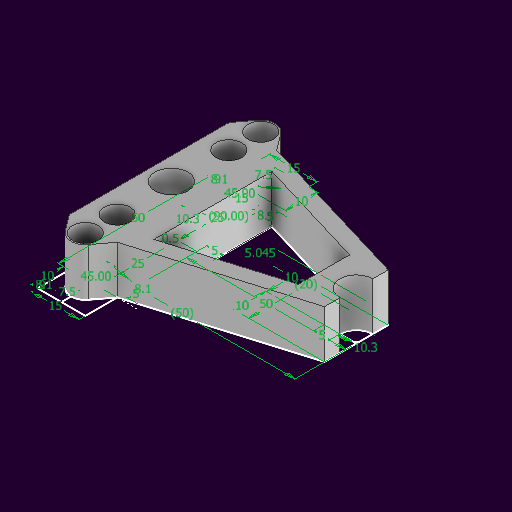
# Autodesk Inventor part: Rod_support_2.1
Saved by Autodesk Inventor 2026.2 (Build 302298000, 298)
## iProperties
Created: 2025-12-19
Part Number: Rod_support_2.1
Material: Generic
Document SubType Name: Modeling
Designer: Cobble
Density: 1 g/cm^3
Appearance: Default
Author: Cobble
Autodesk Inventor part; units mm, degrees
ref_plane "YZ Plane" through (0, 0, 0) normal (1, 0, 0) x (0, 1, 0)
ref_plane "XZ Plane" through (0, 0, 0) normal (0, 1, 0) x (-1, 0, 0)
ref_plane "XY Plane" through (0, 0, 0) normal (0, 0, 1) x (1, 0, 0)
sketch "Sketch1" plane through (0, 0, 0) normal (0, 0, 1) x (1, 0, 0)
  arc A0 (65, 30.15) -> (65, 19.85) centre (65, 25) ccw
  line L0 (65, 30.15) -> (65, 35)
  line L1 (65, 19.85) -> (65, 15)
  line L2 (65, 25) -> (15, 25)
  line L3 (15, 25) -> (15, 50)
  line L4 (15, 25) -> (15, 0)
  line L5 (15, 0) -> (65, 15)
  line L6 (15, 50) -> (65, 35)
  line L7 (15, 50) -> (0, 50)
  line L8 (0, 50) -> (0, 0)
  line L9 (0, 0) -> (15, 0)
  line L10 (15, 25) -> (20, 25)
  line L11 (20, 25) -> (20, 48.5)
  line L12 (20, 25) -> (20, 1.5)
  line L13 (59.85, 25) -> (54.85, 25)
  line L14 (54.85, 25) -> (54.85, 38.045)
  line L15 (54.85, 25) -> (54.85, 11.955)
  line L16 (20, 1.5) -> (20, 6.5)
  line L17 (20, 6.5) -> (54.85, 16.955)
  line L18 (20, 48.5) -> (20, 43.5)
  line L19 (20, 43.5) -> (54.85, 33)
  line L20 (7.5, 50) -> (7.5, 0)
  line L21 (0, 25) -> (15, 25)
  line L22 (0, 50) -> (15, 35)
  line L23 (0, 50) -> (21.2132, 50) construction
  line L24 (0, 0) -> (15, 15)
  line L25 (0, 0) -> (21.2132, 0) construction
  circle A1 centre (7.5, 7.5) radius 4.05
  circle A2 centre (7.5, 42.5) radius 4.05
  line L26 (65, 19.85) -> (65, 25)
  line L27 (65, 30.15) -> (65, 25)
  line L28 (7.5, 25) -> (7, 25)
  circle A3 centre (7, 25) radius 5.15
  line L29 (0, 50) -> (15, 50)
  line L30 (15, 50) -> (15, 60)
  line L31 (15, 60) -> (0, 60)
  line L32 (0, 60) -> (0, 50)
  line L33 (15, 0) -> (0, 0)
  line L34 (0, 0) -> (0, -10)
  line L35 (0, -10) -> (15, -10)
  line L36 (15, -10) -> (15, 0)
  line L37 (7.5, -10) -> (7.5, -2.5)
  line L38 (7.5, 60) -> (7.5, 52.5)
  circle A4 centre (7.5, 52.5) radius 4.05
  circle A5 centre (7.5, 52.5) radius 4.5
  circle A6 centre (7.5, -2.5) radius 4.05
  circle A7 centre (7.5, -2.5) radius 4.5
  line L39 (0, 50) -> (3.9, 55.2)
  line L40 (15, 50) -> (11.1, 55.2)
  line L41 (0, 0) -> (3.9, -5.2)
  line L42 (15, 0) -> (11.1, -5.2)
  point P0 (0, 0)
  point P1 (3.7583, 0)
  point P2 (11.2417, 0)
  point P3 (11.2417, 50)
  point P4 (3.7583, 50)
  point P5 (0, 0)
  dimension "d0" = 10.3
  dimension "d1" = 50
  dimension "d2" = 25
  dimension "d3" = 25
  dimension "d4" = 15
  dimension "d5" = 50
  dimension "d6" = 90
  dimension "d7" = 5
  dimension "d8" = 5
  dimension "d9" = 5
  dimension "d10" = 5
  dimension "d11" = 45
  dimension "d12" = 45
  dimension "d13" = 8.1
  dimension "d14" = 8.1
  dimension "d15" = 50
  dimension "d16" = 10
  dimension "d17" = 20
  dimension "d18" = 10
  dimension "d19" = 5.045
  dimension "d46" = 0.5
  dimension "d47" = 10.3
  dimension "d48" = 15
  dimension "d49" = 10
  dimension "d50" = 15
  dimension "d51" = 10
  dimension "d52" = 7.5
  dimension "d53" = 7.5
  dimension "d54" = 8.1
  dimension "d55" = 9
  dimension "d56" = 8.1
  dimension "d57" = 9
  constraints: 86 end point, 16 point on line, 8 centre point, 8 midpoint, 7 point on circle, 7 vertical, 6 coincident, 6 perpendicular, 5 horizontal, 5 parallel, 4 tangent, 2 equal length, 1 collinear, 1 other
  measures "d0" diameter of A0
  measures "d1" distance of L2.start L4.start
  measures "d2" distance of L4.start L3.end
  measures "d3" distance of L4.start L4.end
  measures "d4" distance of L3.end L8.start
  measures "d5" distance of L8.start L8.end
  measures "d6" angle of L8 L7
  measures "d7" distance of L4.start L12.start
  measures "d8" distance of L13.start L14.start
  measures "d9" distance of L16.start L16.end
  measures "d10" distance of L11.end L18.end
  measures "d11" angle of L22 L23
  measures "d12" angle of L25 L24
  measures "d13" diameter of A1
  measures "d14" diameter of A2
  measures "d15" distance of L4.start point (65, 25)
  measures "d16" distance of L5.end point (65, 25)
  measures "d17" distance of L0.end L5.end
  measures "d18" distance of L0.end point (65, 25)
  measures "d19" distance of L14.end L19.end
  measures "d46" distance of L28.start L28.end
  measures "d47" diameter of A3
  measures "d48" distance of L31.end L30.end
  measures "d49" distance of L30.end L29.end
  measures "d50" distance of L35.end L34.end
  measures "d51" distance of L34.end L33.end
  measures "d52" distance of L37.start L37.end
  measures "d53" distance of L38.start L38.end
  measures "d54" diameter of A4
  measures "d55" diameter of A5
  measures "d56" diameter of A6
  measures "d57" diameter of A7
extrude "Extrusion1" add sketch "Sketch1" along normal blind 15 contours A0 L2 L14 L6 L0 | A0 L1 L5 L15 L2 | L14 L19 L11 L6 | L12 L5 L4 L2 | L2 L3 L6 L11 | L15 L5 L12 L17 | L21 A3 L20 A2 L22 L3 | L4 L24 A1 L20 A3 L21 | L3 L22 A2 L20 A5 L7 | L7 A5 L40 | L4 L9 A7 L20 A1 L24 | A5 L20 A4 L7 | L7 A4 L38 A5 | L42 A7 L9 | A3 L21 L8 L22 A2 L20 | L20 A1 L24 L8 L21 A3 | A5 L7 A4 L20 | L20 A2 L22 L7 A5 | L38 A4 L7 A5 | A7 L37 A6 L9 | L9 A6 L20 A7 | L7 L39 A5 | A7 L9 L24 A1 L20 | L20 A6 L9 A7 | A7 L9 A6 L37 | A7 L41 L9
fillet "Fillet1" radius 2 1 edges at (0, 50, 7.5)
sketch "Sketch2" plane through (0, 0, 0) normal (-1, 0, 0) x (0, 0, 1)
  point P0 (0, 0)
body "Solid1"
